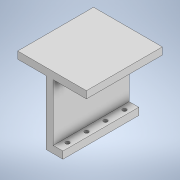
# Autodesk Inventor part: pullyBracket
Saved by Autodesk Inventor 2022.1 (Build 261234020, 234B)
## iProperties
Created: 2021-11-10
Part Number: pullyBracket
Material: Generic
Document SubType Name: Modeling
Designer: robst
Density: 1 g/cm^3
Appearance: Default
Author: robst
Autodesk Inventor part; units mm, degrees
ref_plane "YZ Plane" through (0, 0, 0) normal (1, 0, 0) x (0, 1, 0)
ref_plane "XZ Plane" through (0, 0, 0) normal (0, 1, 0) x (-1, 0, 0)
ref_plane "XY Plane" through (0, 0, 0) normal (0, 0, 1) x (1, 0, 0)
sketch "Sketch1" plane through (0, 0, 0) normal (0, 1, 0) x (-1, 0, 0)
  line L0 (11.2547, 50.8) -> (-11.2547, 50.8)
  line L1 (-11.2547, 50.8) -> (-11.2547, -50.8)
  line L2 (-11.2547, -50.8) -> (11.2547, -50.8)
  line L3 (11.2547, -50.8) -> (11.2547, 50.8)
  line L4 (11.2547, 50.8) -> (-11.2547, -50.8) construction
  line L5 (-11.2547, 50.8) -> (11.2547, -50.8) construction
  point P0 (0, 0)
  dimension "d0" = 101.6
  dimension "d1" = 22.5095
  constraints: 12 end point, 2 midpoint, 2 parallel, 1 horizontal, 1 perpendicular
  measures "d0" distance of L2.end L0.start
  measures "d1" distance of L1.end L2.end
extrude "Extrusion1" add sketch "Sketch1" against normal blind 9.525
sketch "Sketch2" plane through (0, 0, 0) normal (0, 1, 0) x (1, 0, 0)
  line L0 (11.2547, -50.8) -> (-11.2547, -50.8) projected
  line L1 (-11.2547, 50.8) -> (11.2547, 50.8) projected
  line L2 (-11.2547, -50.8) -> (-1.7297, -50.8)
  line L3 (-1.7297, -50.8) -> (-1.7297, 50.8)
  line L4 (-1.7297, 50.8) -> (-11.2547, 50.8)
  line L5 (-11.2547, 50.8) -> (-11.2547, -50.8)
  point P0 (0, 0)
  dimension "d4" = 9.525
  constraints: 8 end point, 2 parallel, 1 horizontal, 1 perpendicular, 1 point on line
  measures "d4" distance between parallel lines of L3 L5
extrude "Extrusion2" add sketch "Sketch2" along normal blind 76.2
sketch "Sketch3" plane through (0, 76.2, 0) normal (0, 1, 0) x (1, 0, 0)
  line L0 (11.2547, -50.8) -> (-11.2547, -50.8) projected
  line L1 (-11.2547, -50.8) -> (-49.3547, -50.8)
  line L2 (-49.3547, -50.8) -> (-49.3547, 50.8)
  line L3 (-49.3547, 50.8) -> (-11.2547, 50.8)
  line L4 (-11.2547, 50.8) -> (-11.2547, -50.8)
  line L5 (-1.7297, -50.8) -> (-1.7297, 50.8) projected
  line L6 (-1.7297, 50.8) -> (-11.2547, 50.8) projected
  line L7 (-11.2547, -50.8) -> (-1.7297, -50.8) projected
  line L8 (11.2547, -50.8) -> (11.2547, 50.8) projected
  line L9 (11.2547, 50.8) -> (-1.7297, 50.8) projected
  line L10 (-11.2547, -50.8) -> (-11.2547, 50.8) projected
  line L11 (-11.2547, -50.8) -> (-1.7297, -50.8)
  line L12 (-1.7297, -50.8) -> (-1.7297, 50.8)
  line L13 (-1.7297, 50.8) -> (-11.2547, 50.8)
  line L14 (-11.2547, 50.8) -> (-11.2547, -50.8)
  line L15 (-1.7297, -50.8) -> (42.7203, -50.8)
  line L16 (42.7203, -50.8) -> (42.7203, 50.8)
  line L17 (42.7203, 50.8) -> (-1.7297, 50.8)
  line L18 (-1.7297, 50.8) -> (-1.7297, -50.8)
  point P0 (0, 0)
  dimension "d7" = 38.1
  dimension "d8" = 44.45
  constraints: 24 end point, 6 parallel, 3 horizontal, 3 perpendicular, 1 point on line
  measures "d7" distance of L2.end L3.end
  measures "d8" distance of L16.end L17.end
extrude "Extrusion3" add sketch "Sketch3" along normal blind 9.525
sketch "Sketch4" plane through (0, 0, 0) normal (0, 1, 0) x (1, 0, 0)
  line L0 (-1.7297, -50.8) -> (11.2547, -50.8) construction
  line L1 (4.7625, -50.8) -> (4.7625, 50.8) construction
  line L2 (-11.2547, 50.8) -> (11.2547, 50.8) construction
  point P0 (0, 0)
  point P1 (4.7625, -38.1)
  point P2 (4.7625, -12.7)
  point P3 (4.7625, 12.7)
  point P4 (4.7625, 38.1)
  dimension "d11" = 12.7
  dimension "d14" = 25.4
  constraints: 2 end point, 2 point on line, 2 vertical, 1 midpoint, 3 other
  measures "d11" distance from line of point (4.763, -38.1) L0
  measures "d14" distance of point (4.763, -38.1) point (4.763, -12.7)
hole "Hole1" at (4.7625, 0, 38.1) at (4.7625, 0, 12.7) at (4.7625, 0, -12.7) at (4.7625, 0, -38.1) direction (0, -1, 0) diameter 5.1054 end through all clearance for "Hex Machine Screw" size "#10" standard "Ansi Unified Screw Threads"
equation "\"d0\" = BaseLength"
equation "\"d1\" = BaseWidth"
equation "\"d2\" = BaseThickness"
equation "\"d4\" = BackWidth"
equation "\"d5\" = BackHeight"
equation "\"d7\" = TopBackExtension"
equation "\"d8\" = TopFrontExtension"
equation "\"d9\" = TopThickness"
equation "\"d11\" = offsetForFirstHole"
equation "\"BaseWidth\" = 22.50948"
equation "\"BaseLength\" = 101.6"
equation "\"BaseThickness\" = 9.525"
equation "\"BackWidth\" = 9.525"
equation "\"BackHeight\" = 76.2"
equation "\"TopBackExtension\" = 38.1"
equation "\"TopFrontExtension\" = 44.45"
equation "\"TopThickness\" = 9.525"
equation "\"offsetForFirstHole\" = 12.7"
body "Solid1"
